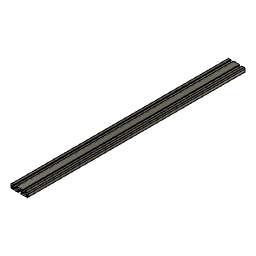
_ProfilStolTeowy40x10_500mm.f1481c84-2a1f-4ead-9c4e-9dfacb96aeeb (Autodesk Fusion 360 design; units mm, degrees)
Autodesk Fusion 360 part; units mm, degrees
sketch "Sketch1" plane through (0, 0, 0) normal (0, 1, 0) x (1, 0, 0)
  line L0 (7.4, -9.8) -> (7.4, -8.7)
  line L1 (0, -10) -> (7.2, -10)
  line L2 (6.9, -8.2) -> (5.2043, -8.2)
  line L3 (4.7932, -7.4154) -> (7.1018, -4.0808)
  line L4 (7.924, -3.65) -> (10, -3.65)
  arc A0 (4.7932, -7.4154) -> (5.2043, -8.2) centre (5.2043, -7.7) ccw
  arc A1 (7.924, -3.65) -> (7.1018, -4.0808) centre (7.924, -4.65) ccw
  arc A2 (7.4, -8.7) -> (6.9, -8.2) centre (6.9, -8.7) ccw
  arc A3 (7.2, -10) -> (7.4, -9.8) centre (7.2, -9.8) ccw
  line L5 (12.6, -9.8) -> (12.6, -8.7)
  arc A4 (12.8982, -4.0808) -> (12.076, -3.65) centre (12.076, -4.65) ccw
  arc A5 (14.7957, -8.2) -> (15.2068, -7.4154) centre (14.7957, -7.7) ccw
  arc A6 (13.1, -8.2) -> (12.6, -8.7) centre (13.1, -8.7) ccw
  line L6 (15.2068, -7.4154) -> (12.8982, -4.0808)
  line L7 (13.1, -8.2) -> (14.7957, -8.2)
  arc A7 (12.6, -9.8) -> (12.8, -10) centre (12.8, -9.8) ccw
  line L8 (12.076, -3.65) -> (10, -3.65)
  line L9 (12.8, -10) -> (18, -10)
  line L10 (20, -8) -> (20, -2)
  circle A8 centre (16.7, -3.3) radius 1.85
  line L11 (16.7, -5.15) -> (17.5637, -5.8434)
  line L12 (18.0081, -4.6081) -> (17.8877, -5.7091)
  arc A9 (17.5637, -5.8434) -> (17.8877, -5.7091) centre (17.6889, -5.6874) ccw
  line L13 (16.7, -3.3) -> (19.7, -3.3) construction
  line L14 (14.85, -3.3) -> (14.1566, -2.4363)
  line L15 (15.3919, -1.9919) -> (14.2909, -2.1123)
  arc A10 (14.2909, -2.1123) -> (14.1566, -2.4363) centre (14.3126, -2.3111) ccw
  line L16 (12.6, -9.8) -> (12.6, -8.7)
  line L17 (16.7, -5.15) -> (17.5637, -5.8434)
  arc A11 (14.2909, -2.1123) -> (14.1566, -2.4363) centre (14.3126, -2.3111) ccw
  circle A12 centre (16.7, -3.3) radius 1.85
  line L18 (12.076, -3.65) -> (10, -3.65)
  arc A13 (14.7957, -8.2) -> (15.2068, -7.4154) centre (14.7957, -7.7) ccw
  line L19 (0, -10) -> (7.2, -10)
  line L20 (18.0081, -4.6081) -> (17.8877, -5.7091)
  line L21 (13.1, -8.2) -> (14.7957, -8.2)
  line L22 (6.9, -8.2) -> (5.2043, -8.2)
  line L23 (14.85, -3.3) -> (14.1566, -2.4363)
  arc A14 (7.924, -3.65) -> (7.1018, -4.0808) centre (7.924, -4.65) ccw
  arc A15 (12.6, -9.8) -> (12.8, -10) centre (12.8, -9.8) ccw
  arc A16 (7.2, -10) -> (7.4, -9.8) centre (7.2, -9.8) ccw
  arc A17 (17.5637, -5.8434) -> (17.8877, -5.7091) centre (17.6889, -5.6874) ccw
  line L24 (15.2068, -7.4154) -> (12.8982, -4.0808)
  arc A18 (12.8982, -4.0808) -> (12.076, -3.65) centre (12.076, -4.65) ccw
  arc A19 (7.4, -8.7) -> (6.9, -8.2) centre (6.9, -8.7) ccw
  arc A20 (4.7932, -7.4154) -> (5.2043, -8.2) centre (5.2043, -7.7) ccw
  line L25 (4.7932, -7.4154) -> (7.1018, -4.0808)
  line L26 (16.7, -3.3) -> (19.7, -3.3) construction
  line L27 (7.4, -9.8) -> (7.4, -8.7)
  line L28 (15.3919, -1.9919) -> (14.2909, -2.1123)
  arc A21 (13.1, -8.2) -> (12.6, -8.7) centre (13.1, -8.7) ccw
  line L29 (7.924, -3.65) -> (10, -3.65)
  line L30 (0, -10) -> (-7.2, -10)
  arc A22 (-7.4, -9.8) -> (-7.2, -10) centre (-7.2, -9.8) ccw
  line L31 (-15.2068, -7.4154) -> (-12.8982, -4.0808)
  arc A23 (-12.8, -10) -> (-12.6, -9.8) centre (-12.8, -9.8) ccw
  line L32 (-15.3919, -1.9919) -> (-14.2909, -2.1123)
  arc A24 (-17.8877, -5.7091) -> (-17.5637, -5.8434) centre (-17.6889, -5.6874) ccw
  line L33 (-14.85, -3.3) -> (-14.1566, -2.4363)
  arc A25 (-12.6, -8.7) -> (-13.1, -8.2) centre (-13.1, -8.7) ccw
  arc A26 (-14.1566, -2.4363) -> (-14.2909, -2.1123) centre (-14.3126, -2.3111) ccw
  line L34 (-16.7, -3.3) -> (-19.7, -3.3) construction
  line L35 (-16.7, -3.3) -> (-19.7, -3.3) construction
  line L36 (-18.0081, -4.6081) -> (-17.8877, -5.7091)
  line L37 (-12.6, -9.8) -> (-12.6, -8.7)
  line L38 (-15.3919, -1.9919) -> (-14.2909, -2.1123)
  line L39 (-18.0081, -4.6081) -> (-17.8877, -5.7091)
  line L40 (-12.6, -9.8) -> (-12.6, -8.7)
  line L41 (-16.7, -5.15) -> (-17.5637, -5.8434)
  line L42 (-12.8, -10) -> (-18, -10)
  arc A27 (-15.2068, -7.4154) -> (-14.7957, -8.2) centre (-14.7957, -7.7) ccw
  line L43 (-4.7932, -7.4154) -> (-7.1018, -4.0808)
  line L44 (-7.4, -9.8) -> (-7.4, -8.7)
  arc A28 (-7.1018, -4.0808) -> (-7.924, -3.65) centre (-7.924, -4.65) ccw
  arc A29 (-5.2043, -8.2) -> (-4.7932, -7.4154) centre (-5.2043, -7.7) ccw
  line L45 (-7.4, -9.8) -> (-7.4, -8.7)
  line L46 (-12.076, -3.65) -> (-10, -3.65)
  arc A30 (-5.2043, -8.2) -> (-4.7932, -7.4154) centre (-5.2043, -7.7) ccw
  line L47 (-14.85, -3.3) -> (-14.1566, -2.4363)
  arc A31 (-14.1566, -2.4363) -> (-14.2909, -2.1123) centre (-14.3126, -2.3111) ccw
  arc A32 (-12.076, -3.65) -> (-12.8982, -4.0808) centre (-12.076, -4.65) ccw
  line L48 (-15.2068, -7.4154) -> (-12.8982, -4.0808)
  circle A33 centre (-16.7, -3.3) radius 1.85
  line L49 (-16.7, -5.15) -> (-17.5637, -5.8434)
  line L50 (-20, -8) -> (-20, -2)
  arc A34 (-15.2068, -7.4154) -> (-14.7957, -8.2) centre (-14.7957, -7.7) ccw
  arc A35 (-12.8, -10) -> (-12.6, -9.8) centre (-12.8, -9.8) ccw
  arc A36 (-12.6, -8.7) -> (-13.1, -8.2) centre (-13.1, -8.7) ccw
  circle A37 centre (-16.7, -3.3) radius 1.85
  line L51 (-13.1, -8.2) -> (-14.7957, -8.2)
  arc A38 (-17.8877, -5.7091) -> (-17.5637, -5.8434) centre (-17.6889, -5.6874) ccw
  arc A39 (-12.076, -3.65) -> (-12.8982, -4.0808) centre (-12.076, -4.65) ccw
  line L52 (-7.924, -3.65) -> (-10, -3.65)
  line L53 (0, -10) -> (-7.2, -10)
  line L54 (-4.7932, -7.4154) -> (-7.1018, -4.0808)
  line L55 (-12.076, -3.65) -> (-10, -3.65)
  arc A40 (-6.9, -8.2) -> (-7.4, -8.7) centre (-6.9, -8.7) ccw
  line L56 (-6.9, -8.2) -> (-5.2043, -8.2)
  line L57 (-6.9, -8.2) -> (-5.2043, -8.2)
  line L58 (-13.1, -8.2) -> (-14.7957, -8.2)
  arc A41 (-7.4, -9.8) -> (-7.2, -10) centre (-7.2, -9.8) ccw
  arc A42 (-7.1018, -4.0808) -> (-7.924, -3.65) centre (-7.924, -4.65) ccw
  arc A43 (-6.9, -8.2) -> (-7.4, -8.7) centre (-6.9, -8.7) ccw
  line L59 (-7.924, -3.65) -> (-10, -3.65)
  arc A44 (2.6, -1.3) -> (3.1, -1.8) centre (3.1, -1.3) ccw
  line L60 (-5.2068, -2.5846) -> (-2.8982, -5.9192)
  arc A45 (2.076, -6.35) -> (2.8982, -5.9192) centre (2.076, -5.35) ccw
  line L61 (2.076, -6.35) -> (0, -6.35)
  line L62 (2.076, -6.35) -> (0, -6.35)
  arc A46 (5.2068, -2.5846) -> (4.7957, -1.8) centre (4.7957, -2.3) ccw
  arc A47 (-2.8982, -5.9192) -> (-2.076, -6.35) centre (-2.076, -5.35) ccw
  arc A48 (-3.1, -1.8) -> (-2.6, -1.3) centre (-3.1, -1.3) ccw
  arc A49 (2.8, 0) -> (2.6, -0.2) centre (2.8, -0.2) ccw
  arc A50 (-2.6, -0.2) -> (-2.8, 0) centre (-2.8, -0.2) ccw
  arc A51 (2.8, 0) -> (2.6, -0.2) centre (2.8, -0.2) ccw
  arc A52 (-2.8982, -5.9192) -> (-2.076, -6.35) centre (-2.076, -5.35) ccw
  arc A53 (-2.6, -0.2) -> (-2.8, 0) centre (-2.8, -0.2) ccw
  line L63 (-3.1, -1.8) -> (-4.7957, -1.8)
  line L64 (-2.076, -6.35) -> (0, -6.35)
  arc A54 (2.076, -6.35) -> (2.8982, -5.9192) centre (2.076, -5.35) ccw
  line L65 (-2.6, -0.2) -> (-2.6, -1.3)
  arc A55 (2.6, -1.3) -> (3.1, -1.8) centre (3.1, -1.3) ccw
  line L66 (3.1, -1.8) -> (4.7957, -1.8)
  arc A56 (-3.1, -1.8) -> (-2.6, -1.3) centre (-3.1, -1.3) ccw
  line L67 (2.6, -0.2) -> (2.6, -1.3)
  arc A57 (-4.7957, -1.8) -> (-5.2068, -2.5846) centre (-4.7957, -2.3) ccw
  line L68 (-2.076, -6.35) -> (0, -6.35)
  line L69 (2.6, -0.2) -> (2.6, -1.3)
  line L70 (5.2068, -2.5846) -> (2.8982, -5.9192)
  line L71 (-2.6, -0.2) -> (-2.6, -1.3)
  line L72 (-18, 0) -> (-2.8, 0)
  line L73 (2.8, 0) -> (18, 0)
  arc A58 (-20, -8) -> (-18, -10) centre (-18, -8) ccw
  arc A59 (-18, 0) -> (-20, -2) centre (-18, -2) ccw
  arc A60 (18, -10) -> (20, -8) centre (18, -8) ccw
  arc A61 (20, -2) -> (18, 0) centre (18, -2) ccw
  point P0 (20, 0)
  point P1 (7.4, -8.2)
  point P2 (4.25, -8.2)
  point P3 (15.75, -8.2)
  point P4 (12.6, -8.2)
  point P5 (17.8481, -6.0716)
  point P6 (13.9284, -2.1519)
  point P7 (17.8481, -6.0716)
  point P8 (12.6, -8.2)
  point P9 (4.25, -8.2)
  point P10 (15.75, -8.2)
  point P11 (7.4, -8.2)
  point P12 (13.9284, -2.1519)
  point P13 (-4.25, -8.2)
  point P14 (-17.8481, -6.0716)
  point P15 (-17.8481, -6.0716)
  point P16 (-4.25, -8.2)
  point P17 (-7.4, -8.2)
  point P18 (-15.75, -8.2)
  point P19 (-12.6, -8.2)
  point P20 (-13.9284, -2.1519)
  point P21 (-7.4, -8.2)
  point P22 (-13.9284, -2.1519)
  point P23 (-12.6, -8.2)
  point P24 (-15.75, -8.2)
  point P25 (-5.75, -8.2)
  point P26 (4.85, -3.3)
  point P27 (4.85, -3.3)
  point P28 (-5.75, -8.2)
  point P29 (-2.6, -1.8)
  point P30 (-2.6, -1.8)
  point P31 (2.6, -1.8)
  point P32 (2.6, -1.8)
  dimension "d1" = 20
  dimension "d2" = 10
  dimension "d5" = 3.15
  dimension "d7" = 0.5
  dimension "d8" = 1
  dimension "d9" = 0.5
  dimension "d10" = 0.2
  dimension "d13" = 3.7
  dimension "d16" = 3
  dimension "d17" = 0.2
  dimension "d20" = 3
  dimension "d21" = 0.2
  dimension "d23" = 10
  dimension "d24" = 3.15
  dimension "d25" = 0.5
  dimension "d26" = 1
  dimension "d27" = 0.5
  dimension "d28" = 0.2
  dimension "d29" = 3.7
  dimension "d30" = 3
  dimension "d31" = 0.2
  dimension "d32" = 3
  dimension "d33" = 0.2
  dimension "d44" = 2
  dimension "d45" = 2
  dimension "d46" = 2
  dimension "d47" = 2
  constraint vertical L0
  constraint perpendicular L0 L2
  constraint coincident P9 L2
  constraint coincident P9 L3
  constraint tangent L2 A0
  constraint tangent L3 A0
  constraint tangent L3 A1
  constraint tangent L4 A1
  constraint coincident P11 L0
  constraint coincident P11 L2
  constraint tangent L0 A2
  constraint tangent L2 A2
  constraint tangent L0 A3
  constraint tangent L1 A3
  constraint tangent A7 L9
  constraint coincident A8 L11.start
  constraint coincident P7 L11
  constraint coincident P7 L12
  constraint tangent L11 A9
  constraint tangent L12 A9
  constraint coincident A8 L14.start
  constraint horizontal L13
  constraint coincident A8.centre L13.start
  constraint coincident P12 L14
  constraint coincident P12 L15
  constraint tangent L14 A10
  constraint tangent L15 A10
  constraint vertical L27
  constraint perpendicular L22 L27
  constraint coincident P9 L22
  constraint coincident P9 L25
  constraint tangent L22 A20
  constraint tangent A20 L25
  constraint tangent A14 L25
  constraint tangent A14 L29
  constraint coincident P11 L27
  constraint coincident P11 L22
  constraint tangent A19 L27
  constraint tangent L22 A19
  constraint tangent A16 L27
  constraint tangent L19 A16
  constraint coincident L11.start A12
  constraint coincident P7 L17
  constraint coincident P7 L20
  constraint tangent L17 A17
  constraint tangent L20 A17
  constraint coincident L14.start A12
  constraint horizontal L26
  constraint coincident P12 L23
  constraint coincident P12 L28
  constraint tangent A11 L23
  constraint tangent A11 L28
  constraint tangent A53 L72
  constraint tangent A49 L73
  constraint tangent L42 A58
  constraint tangent L50 A58
  constraint tangent L50 A59
  constraint tangent L72 A59
  constraint tangent L9 A60
  constraint tangent L10 A60
  constraint coincident P0 L10
  constraint coincident P0 L73
  constraint tangent L10 A61
  constraint tangent L73 A61
  measures "d1" distance of origin P0
  measures "d2" distance of origin L1.start
  measures "d5" distance of P11 P9
  measures "d7" radius of A0
  measures "d8" radius of A1
  measures "d9" radius of A2
  measures "d10" radius of A3
  measures "d13" diameter of A8
  measures "d16" distance of A8.centre P7
  measures "d17" radius of A9
  measures "d20" distance of A8.centre P12
  measures "d21" radius of A10
  measures "d23" distance of L1.start origin
  measures "d24" distance of P9 P11
  measures "d25" radius of A20
  measures "d26" radius of A14
  measures "d27" radius of A19
  measures "d28" radius of A16
  measures "d29" diameter of A12
  measures "d30" distance of A8.centre P7
  measures "d31" radius of A17
  measures "d32" distance of A8.centre P12
  measures "d33" radius of A11
  measures "d44" radius of A58
  measures "d45" radius of A59
  measures "d46" radius of A60
  measures "d47" radius of A61
extrude "Extrude1" add sketch "Sketch1" along normal blind 500
sketch "Sketch2" plane through (0, 0, 3.65) normal (0, 0, 1) x (-1, 0, 0)
  line L0 (12.076, 0) -> (7.924, 0)
  line L1 (7.924, 0) -> (7.924, -500)
  line L2 (7.924, -500) -> (12.076, -500)
  line L3 (12.076, -500) -> (12.076, 0)
  line L4 (10, 0) -> (10, -50)
  circle A0 centre (10, -50) radius 1.5
  circle A1 centre (-10, -50) radius 1.5
  circle A2 centre (10, -100) radius 1.5
  circle A3 centre (-10, -100) radius 1.5
  circle A4 centre (10, -150) radius 1.5
  circle A5 centre (-10, -150) radius 1.5
  circle A6 centre (10, -200) radius 1.5
  circle A7 centre (-10, -200) radius 1.5
  circle A8 centre (10, -250) radius 1.5
  circle A9 centre (-10, -250) radius 1.5
  circle A10 centre (10, -300) radius 1.5
  circle A11 centre (-10, -300) radius 1.5
  circle A12 centre (10, -350) radius 1.5
  circle A13 centre (-10, -350) radius 1.5
  circle A14 centre (10, -400) radius 1.5
  circle A15 centre (-10, -400) radius 1.5
  circle A16 centre (10, -450) radius 1.5
  circle A17 centre (-10, -450) radius 1.5
  dimension "d52" = -20
  dimension "d53" = -400
  constraint midpoint L0 L4.start
  constraint perpendicular L0 L4
  constraint coincident L4.end A0.centre
extrude "Extrude2" cut sketch "Sketch2" against normal blind 4 contours A0 | A1 | A2 | A3 | A4 | A5 | A6 | A7 | A8 | A9 | A10 | A11 | A12 | A13 | A14 | A15 | A16 | A17
chamfer "Chamfer1" distance 1 angle 45 6 edges at (-8.6015, 449.4576, 3.65) (11.3985, 449.4576, 3.65) (-8.6015, 399.4576, 3.65) (11.3985, 399.4576, 3.65) (-8.6015, 349.4576, 3.65) (11.3985, 349.4576, 3.65)
chamfer "Chamfer2" distance 1 angle 45 12 edges at (-8.6015, 299.4576, 3.65) (11.3985, 299.4576, 3.65) (-8.6015, 249.4576, 3.65) (11.3985, 249.4576, 3.65) (-8.6015, 199.4576, 3.65) (11.3985, 199.4576, 3.65) (-8.6015, 149.4576, 3.65) (11.3985, 149.4576, 3.65) (-8.6015, 99.4576, 3.65) (11.3985, 99.4576, 3.65) (-8.6015, 49.4576, 3.65) (11.3985, 49.4576, 3.65)
